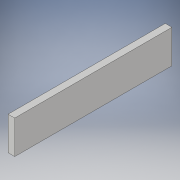
# Autodesk Inventor part: Outboard wing brace
Saved by Autodesk Inventor 2018 (Build 220112000, 112)
## iProperties
Created: 2018-08-13
Part Number: Outboard wing brace
Material: Generic
Document SubType Name: Modeling
Designer: Michael Gunderman
Density: 1 g/cm^3
Appearance: Default
Author: Michael Gunderman
Autodesk Inventor part; units mm, degrees
ref_plane "YZ Plane" through (0, 0, 0) normal (1, 0, 0) x (0, 1, 0)
ref_plane "XZ Plane" through (0, 0, 0) normal (0, 1, 0) x (-1, 0, 0)
ref_plane "XY Plane" through (0, 0, 0) normal (0, 0, 1) x (1, 0, 0)
sketch "Sketch1" plane through (0, 0, 0) normal (1, 0, 0) x (0, 1, 0)
  line L0 (0, 0) -> (35, 0)
  line L1 (35, 0) -> (35, -165)
  line L2 (35, -165) -> (0, -165)
  line L3 (0, -165) -> (0, 0)
  dimension "d0" = 35
  dimension "d1" = 165
  constraints: 8 end point, 2 perpendicular, 1 horizontal, 1 vertical
  measures "d0" distance of L0.start L0.end
  measures "d1" distance of L0.end L1.end
extrude "Extrusion1" add sketch "Sketch1" against normal blind 7
body "Solid1"
